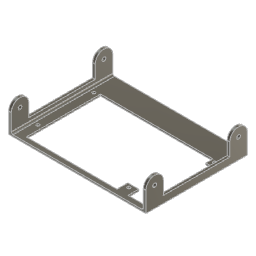
ATX Power Supply Mount v5 (Autodesk Fusion 360 design; units mm, degrees)
Autodesk Fusion 360 part; units mm, degrees
note: some values were not read from the file. Chosen so that the rebuilt part matches the saved one: which face or edge a step refers to.
sketch "Sketch1" plane through (0, 0, 0) normal (0, 0, 1) x (1, 0, 0)
  line L0 (114, 0) -> (114, 6)
  circle A0 centre (114, 6) radius 1.75
  circle A1 centre (0, 16) radius 1.75
  circle A2 centre (0, 80) radius 1.75
  line L1 (108.781, -2.4453) -> (5.219, 82.4453) construction
  line L2 (5.219, -2.4453) -> (108.781, 82.4453) construction
  line L3 (0, 80) -> (138, 80)
  circle A3 centre (138, 80) radius 1.75
  line L4 (69, 80) -> (69, 95.6293)
  line L5 (69, 80) -> (69, 0)
  line L6 (147.5, -8) -> (-9.5, -8)
  line L7 (-9.5, -8) -> (-9.5, 88)
  line L8 (-9.5, 88) -> (147.5, 88)
  line L9 (147.5, 88) -> (147.5, -8)
  line L10 (147.5, -8) -> (-9.5, 88) construction
  line L11 (-9.5, -8) -> (147.5, 88) construction
  line L12 (5.219, 82.4453) -> (108.781, 82.4453)
  line L13 (108.781, 82.4453) -> (108.781, -2.4453)
  line L14 (108.781, -2.4453) -> (5.219, -2.4453)
  line L15 (5.219, -2.4453) -> (5.219, 82.4453)
  line L16 (108.781, 82.4453) -> (133.6988, 82.4453)
  line L17 (133.6988, 82.4453) -> (133.6988, 10.0014)
  line L18 (133.6988, 10.0014) -> (108.781, 10.0014)
  line L19 (108.781, 10.0014) -> (108.781, 82.4453)
  line L20 (133.6988, 74.3424) -> (139.733, 74.3424)
  line L21 (139.733, 74.3424) -> (139.733, -2.1342)
  line L22 (139.733, -2.1342) -> (133.6988, -2.1342)
  line L23 (133.6988, -2.1342) -> (133.6988, 74.3424)
  line L24 (133.6988, -2.1342) -> (121.2399, -2.1342)
  line L25 (121.2399, -2.1342) -> (121.2399, 10.0014)
  line L26 (121.2399, 10.0014) -> (133.6988, 10.0014)
  line L27 (133.6988, 10.0014) -> (133.6988, -2.1342)
  point P0 (57, 40)
  point P1 (57, 40)
  point P2 (69, 40)
  dimension "d1" = 114
  dimension "d2" = 6
  dimension "d3" = 16
  dimension "d4" = 64
  dimension "d6" = 3.5
  dimension "d8" = 3.5
  dimension "d9" = 3.5
  dimension "d12" = 138
  dimension "d13" = 3.5
  dimension "d14" = 80
  dimension "d15" = 157
  dimension "d16" = 96
  constraint coincident L0.end A0.centre
  constraint coincident L1 P1
  constraint coincident L2 P1
  constraint coincident P1 P0
  constraint coincident A2.centre L3.start
  constraint horizontal L3
  constraint coincident L3.end A3.centre
  constraint midpoint L3 L4.start
  constraint perpendicular L3 L5
  constraint horizontal L6
  constraint perpendicular L6 L7
  constraint parallel L6 L8
  constraint parallel L7 L9
  constraint coincident L10 P2
  constraint coincident L11 P2
  constraint midpoint L5 P2
  constraint horizontal L12
  constraint vertical L13
  constraint horizontal L14
  constraint vertical L15
  constraint horizontal L16
  constraint vertical L17
  constraint horizontal L18
  constraint vertical L19
  constraint horizontal L20
  constraint vertical L21
  constraint horizontal L22
  constraint vertical L23
  constraint coincident L17 L20.start
  constraint horizontal L24
  constraint vertical L25
  constraint horizontal L26
  constraint vertical L27
  constraint midpoint L18 L25.end
  measures "d1" distance of origin L0.start
  measures "d2" distance of L0.start L0.end
  measures "d3" distance of origin A1.centre
  measures "d4" distance of A1.centre A2.centre
  measures "d6" diameter of A0
  measures "d8" diameter of A1
  measures "d9" diameter of A2
  measures "d12" distance of A2.centre L3.end
  measures "d13" diameter of A3
  measures "d14" distance of L4.start L5.end
  measures "d15" distance of L7.end L8.end
  measures "d16" distance of L6.end L7.end
extrude "Extrude1" add sketch "Sketch1" along normal blind 2 contours L17 L20 L21 L22 L23 L27 | L18 L23 L24 L25 L26 L27 | L6 L7 L8 L9
extrude "Extrude2" cut sketch "Sketch1" along normal blind 2 contours L17 L20 L21 L22 L23 L27 | L18 L23 L24 L25 L26 L27
sketch "Sketch4" plane through (0, 0, 2) normal (0, 0, 1) x (-1, 0, 0)
  line L0 (-121.2399, 2.1342) -> (-121.2399, -10.0014)
  line L1 (-121.2399, -10.0014) -> (-108.781, -10.0014)
  line L2 (-108.781, -10.0014) -> (-108.781, 2.4453)
  line L3 (-108.781, 2.4453) -> (-5.219, 2.4453)
  line L4 (-5.219, 2.4453) -> (-5.219, -82.4453)
  line L5 (-5.219, -82.4453) -> (-133.6988, -82.4453)
  line L6 (-133.6988, -82.4453) -> (-133.6988, -74.3424)
  line L7 (-133.6988, -74.3424) -> (-139.733, -74.3424)
  line L8 (-139.733, -74.3424) -> (-139.733, 2.1342)
  line L9 (-139.733, 2.1342) -> (-121.2399, 2.1342)
  circle A0 centre (-114, -6) radius 1.75
  circle A1 centre (0, -16) radius 1.75
  circle A2 centre (0, -80) radius 1.75
  circle A3 centre (-138, -80) radius 1.75
  line L10 (-147.5, -88) -> (9.5, -88)
  line L11 (9.5, -88) -> (9.5, 8)
  line L12 (9.5, 8) -> (-147.5, 8)
  line L13 (-147.5, 8) -> (-147.5, -88)
sketch "Sketch5" plane through (0, 0, 0) normal (0, 0, -1) x (1, 0, 0)
  line L0 (139.733, -74.3424) -> (133.6988, -74.3424)
  line L1 (133.6988, -74.3424) -> (133.6988, -82.4453)
  line L2 (133.6988, -82.4453) -> (5.219, -82.4453)
  line L3 (5.219, -82.4453) -> (5.219, 2.4453)
  line L4 (5.219, 2.4453) -> (108.781, 2.4453)
  line L5 (108.781, 2.4453) -> (108.781, -10.0014)
  line L6 (108.781, -10.0014) -> (121.2399, -10.0014)
  line L7 (121.2399, -10.0014) -> (121.2399, 2.1342)
  line L8 (121.2399, 2.1342) -> (139.733, 2.1342)
  line L9 (139.733, 2.1342) -> (139.733, -74.3424)
  circle A0 centre (114, -6) radius 1.75
  circle A1 centre (0, -16) radius 1.75
  circle A2 centre (0, -80) radius 1.75
  circle A3 centre (138, -80) radius 1.75
  line L10 (-9.5, -88) -> (147.5, -88)
  line L11 (147.5, -88) -> (147.5, 8)
  line L12 (147.5, 8) -> (-9.5, 8)
  line L13 (-9.5, 8) -> (-9.5, -88)
  line L14 (147.5, 8) -> (144.5, 8)
  line L15 (144.5, 8) -> (144.5, -88)
  line L16 (144.5, -88) -> (147.5, -88)
  line L17 (147.5, -88) -> (147.5, 8)
  line L18 (-9.5, -88) -> (-6.5, -88)
  line L19 (-6.5, -88) -> (-6.5, 8)
  line L20 (-6.5, 8) -> (-9.5, 8)
  line L21 (-9.5, 8) -> (-9.5, -88)
  line L22 (-6.5, 8) -> (-9.5, 8)
  line L23 (-9.5, 8) -> (-9.5, -108)
  line L24 (-9.5, -108) -> (-6.5, -108)
  line L25 (-6.5, -108) -> (-6.5, 8)
  line L26 (147.5, 8) -> (144.5, 8)
  line L27 (144.5, 8) -> (144.5, -108)
  line L28 (144.5, -108) -> (147.5, -108)
  line L29 (147.5, -108) -> (147.5, 8)
  dimension "d21" = 3
  dimension "d22" = 3
  dimension "d41" = 116
  dimension "d42" = 116
  constraint horizontal L14
  constraint vertical L15
  constraint horizontal L16
  constraint vertical L17
  constraint coincident L11.end L12.start
  constraint horizontal L18
  constraint vertical L19
  constraint horizontal L20
  constraint vertical L21
  constraint coincident L10.start L13.end
  constraint horizontal L22
  constraint vertical L23
  constraint horizontal L24
  constraint vertical L25
  constraint horizontal L26
  constraint vertical L27
  constraint horizontal L28
  constraint vertical L29
  measures "d21" distance of L11.end L14.end
  measures "d22" distance of L10.start L18.end
  measures "d41" distance of L19.end L24.end
  measures "d42" distance of L11.end L28.end
extrude "Extrude6" add 1 faces at (42.8333, 88, 0.6667) along direction (0, 1, 0) blind 20
extrude "Extrude7" add sketch "Sketch5" against normal blind 8 contours L10 L12 L13 L18 L19 L20 L21 L22 L23 L25 | L10 L18 L23 L24 L25 | L10 L11 L12 L14 L15 L16 L17 L26 L27 L29 | L10 L16 L27 L28 L29
sketch "Sketch9" plane through (0, 0, 8) normal (0, 0, 1) x (-1, 0, 0)
  line L0 (6.5, 8) -> (6.5, -108)
  line L1 (6.5, -108) -> (9.5, -108)
  line L2 (9.5, -108) -> (9.5, 8)
  line L3 (9.5, 8) -> (6.5, 8)
  line L4 (6.5, 8) -> (9.5, 8)
  line L5 (9.5, 8) -> (9.5, -12)
  line L6 (9.5, -12) -> (6.5, -12)
  line L7 (6.5, -12) -> (6.5, 8)
  line L8 (9.5, -108) -> (6.5, -108)
  line L9 (6.5, -108) -> (6.5, -88)
  line L10 (6.5, -88) -> (9.5, -88)
  line L11 (9.5, -88) -> (9.5, -108)
  dimension "d45" = 20
  dimension "d46" = 20
  constraint horizontal L4
  constraint vertical L5
  constraint horizontal L6
  constraint vertical L7
  constraint coincident L0.start L3.end
  constraint horizontal L8
  constraint vertical L9
  constraint horizontal L10
  constraint vertical L11
  constraint coincident L1.end L2.start
  measures "d45" distance of L0.start L6.end
  measures "d46" distance of L1.end L10.end
sketch "Sketch10" plane through (0, 0, 8) normal (0, 0, 1) x (-1, 0, 0)
  line L0 (-147.5, 8) -> (-147.5, -108)
  line L1 (-147.5, -108) -> (-144.5, -108)
  line L2 (-144.5, -108) -> (-144.5, 8)
  line L3 (-144.5, 8) -> (-147.5, 8)
  line L4 (-144.5, -108) -> (-147.5, -108)
  line L5 (-147.5, -108) -> (-147.5, -88)
  line L6 (-147.5, -88) -> (-144.5, -88)
  line L7 (-144.5, -88) -> (-144.5, -108)
  line L8 (-147.5, 8) -> (-144.5, 8)
  line L9 (-144.5, 8) -> (-144.5, -12)
  line L10 (-144.5, -12) -> (-147.5, -12)
  line L11 (-147.5, -12) -> (-147.5, 8)
  dimension "d47" = 20
  dimension "d48" = 3
  dimension "d49" = 20
  constraint horizontal L4
  constraint vertical L5
  constraint horizontal L6
  constraint vertical L7
  constraint coincident L1.end L2.start
  constraint horizontal L8
  constraint vertical L9
  constraint horizontal L10
  constraint vertical L11
  constraint coincident L0.start L3.end
  measures "d47" distance of L1.end L6.end
  measures "d48" distance of L0.start L2.end
  measures "d49" distance of L0.start L10.end
extrude "Extrude8" add sketch "Sketch10" sketch "Sketch9" along normal blind 25 contours L0 L2 L3 L8 L9 L10 L11 | L0 L1 L2 L4 L5 L6 L7 of sketch 2 contours L0 L2 L3 L4 L5 L6 L7 | L0 L1 L2 L8 L9 L10 L11
sketch "Sketch11" plane through (147.5, 0, 0) normal (1, 0, 0) x (0, 1, 0)
  line L0 (-8, 0) -> (108, 0)
  line L1 (108, 0) -> (108, 33)
  line L2 (108, 33) -> (88, 33)
  line L3 (88, 33) -> (88, 8)
  line L4 (88, 8) -> (12, 8)
  line L5 (12, 8) -> (12, 33)
  line L6 (12, 33) -> (-8, 33)
  line L7 (-8, 33) -> (-8, 0)
  line L8 (-8, 33) -> (12, 33)
  line L9 (12, 33) -> (12, 13)
  line L10 (12, 13) -> (-8, 13)
  line L11 (-8, 13) -> (-8, 33)
  line L12 (88, 33) -> (108, 33)
  line L13 (108, 33) -> (108, 13)
  line L14 (108, 13) -> (88, 13)
  line L15 (88, 13) -> (88, 33)
  circle A0 centre (98, 23) radius 2.15
  circle A1 centre (2, 23) radius 2.15
  dimension "d52" = 20
  dimension "d53" = 20
  dimension "d54" = 4.3
  dimension "d55" = 4.3
  constraint horizontal L8
  constraint vertical L9
  constraint horizontal L10
  constraint vertical L11
  constraint coincident L6.end L7.start
  constraint horizontal L12
  constraint vertical L13
  constraint horizontal L14
  constraint vertical L15
  constraint coincident L2.end L3.start
  measures "d52" distance of L6.end L10.end
  measures "d53" distance of L2.end L14.end
  measures "d54" diameter of A0
  measures "d55" diameter of A1
extrude "Extrude9" cut sketch "Sketch11" against normal blind 157 contours A0 | A1
fillet "Fillet2" radius 10 8 edges at (-8, -8, 33) (-8, 12, 33) (-8, 88, 33) (-8, 108, 33) (146, -8, 33) (146, 12, 33) (146, 88, 33) (146, 108, 33)
fillet "Fillet3" radius 2 2 edges at (144.5, 50, 2) (-6.5, 50, 2)
extrude "Extrude3" [rolled back] along distance 5 taper angle 0
sketch "Sketch6" plane through (0, 0, -5) normal (0, 0, -1) x (1, 0, 0)
  line L0 (-9.5, 8) -> (-9.5, -88)
  line L1 (-9.5, -88) -> (-6.5, -88)
  line L2 (-6.5, -88) -> (-6.5, 8)
  line L3 (-6.5, 8) -> (-9.5, 8)
  line L4 (-9.5, 8) -> (-6.5, 8)
  line L5 (-6.5, 8) -> (-6.5, -12)
  line L6 (-6.5, -12) -> (-9.5, -12)
  line L7 (-9.5, -12) -> (-9.5, 8)
  line L8 (-9.5, -88) -> (-6.5, -88)
  line L9 (-6.5, -88) -> (-6.5, -68)
  line L10 (-6.5, -68) -> (-9.5, -68)
  line L11 (-9.5, -68) -> (-9.5, -88)
  dimension "d25" = 20
  dimension "d26" = 3
  dimension "d27" = 20
  constraint horizontal L4
  constraint vertical L5
  constraint horizontal L6
  constraint vertical L7
  constraint coincident L0.start L3.end
  constraint horizontal L8
  constraint vertical L9
  constraint horizontal L10
  constraint vertical L11
  constraint coincident L0.end L1.start
  measures "d25" distance of L0.start L6.end
  measures "d26" distance of L0.end L1.end
  measures "d27" distance of L0.end L10.end
sketch "Sketch7" plane through (0, 0, -5) normal (0, 0, -1) x (1, 0, 0)
  line L0 (147.5, -88) -> (147.5, 8)
  line L1 (147.5, 8) -> (144.5, 8)
  line L2 (144.5, 8) -> (144.5, -88)
  line L3 (144.5, -88) -> (147.5, -88)
  line L4 (144.5, 8) -> (147.5, 8)
  line L5 (147.5, 8) -> (147.5, -12)
  line L6 (147.5, -12) -> (144.5, -12)
  line L7 (144.5, -12) -> (144.5, 8)
  line L8 (144.5, -88) -> (147.5, -88)
  line L9 (147.5, -88) -> (147.5, -68)
  line L10 (147.5, -68) -> (144.5, -68)
  line L11 (144.5, -68) -> (144.5, -88)
  dimension "d28" = 20
  dimension "d29" = 3
  dimension "d30" = 20
  constraint horizontal L4
  constraint vertical L5
  constraint horizontal L6
  constraint vertical L7
  constraint coincident L1.end L2.start
  constraint horizontal L8
  constraint vertical L9
  constraint horizontal L10
  constraint vertical L11
  constraint coincident L2.end L3.start
  measures "d28" distance of L1.end L6.end
  measures "d29" distance of L2.end L0.start
  measures "d30" distance of L2.end L10.end
extrude "Extrude4" [rolled back] along distance 15 taper angle 0
sketch "Sketch8" plane through (147.5, 0, 0) normal (1, 0, 0) x (0, 1, 0)
  line L0 (88, -20) -> (88, 2)
  line L1 (88, 2) -> (-8, 2)
  line L2 (-8, 2) -> (-8, -20)
  line L3 (-8, -20) -> (12, -20)
  line L4 (12, -20) -> (12, -5)
  line L5 (12, -5) -> (68, -5)
  line L6 (68, -5) -> (68, -20)
  line L7 (68, -20) -> (88, -20)
  circle A0 centre (2, -12.5) radius 2.2
  circle A1 centre (78, -12.5) radius 2.2
  dimension "d33" = 4.4
  dimension "d34" = 4.4
  measures "d33" diameter of A0
  measures "d34" diameter of A1
extrude "Extrude5" [rolled back] along distance -157 taper angle 0
fillet "Fillet1" [rolled back] radius 10
